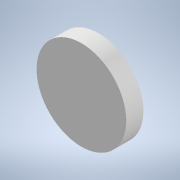
# Autodesk Inventor part: WheelMod6
Saved by Autodesk Inventor 2020 (Build 240168000, 168)
## iProperties
Created: 2020-01-19
Part Number: WheelMod6
Material: Generic
Document SubType Name: Modeling
Designer: srini
Density: 1 g/cm^3
Appearance: Default
Author: srini
Autodesk Inventor part; units mm, degrees
ref_plane "YZ Plane" through (0, 0, 0) normal (1, 0, 0) x (0, 1, 0)
ref_plane "XZ Plane" through (0, 0, 0) normal (0, 1, 0) x (-1, 0, 0)
sketch "Sketch1" plane through (0, 0, 0) normal (0, 0, 1) x (1, 0, 0)
  circle A0 centre (66.294, 0) radius 66.3424 projected
  point P0 (0, 0)
ref_plane "Work Plane1" through (-7.8739, -74.1679, -25.4) normal (0, 0, -1) x (0, 1, 0)
extrude "Extrusion1" add sketch "Sketch1" against normal up to surface (25.4 mm away)
body "Solid1"
